Autodesk Inventor part; units mm, degrees
(part 2 of 2)
sketch "Sketch17" plane through (0, 22.225, 0) normal (0, 1, 0) x (1, 0, 0)
  line L0 (-762.5068, 1886.6652) -> (209.7128, 1886.6652) construction
  line L1 (209.7128, 1886.6652) -> (209.7128, -25.5438) construction
  line L2 (209.7128, -25.5438) -> (-762.5068, -25.5438) construction
  line L3 (-762.5068, -25.5438) -> (-762.5068, 1886.6652) construction
  line L4 (-762.5068, 1886.6652) -> (209.7128, 1886.6652) construction
  line L5 (209.7128, 1886.6652) -> (209.7128, -25.5438) construction
  line L6 (209.7128, -25.5438) -> (-762.5068, -25.5438) construction
  line L7 (-762.5068, -25.5438) -> (-762.5068, 1886.6652) construction
  point P0 (0, 0)
  point P1 (0, 0)
  point P2 (0, 0)
  constraints: 4 other
decal "Decal2"
sketch "Sketch18" plane through (0, 22.225, 0) normal (0, 1, 0) x (1, 0, 0)
  line L0 (-762.5068, 1886.6652) -> (209.7128, 1886.6652) construction
  line L1 (209.7128, 1886.6652) -> (209.7128, -25.5438) construction
  line L2 (209.7128, -25.5438) -> (-762.5068, -25.5438) construction
  line L3 (-762.5068, -25.5438) -> (-762.5068, 1886.6652) construction
  line L4 (-762.5068, 1886.6652) -> (209.7128, 1886.6652) construction
  line L5 (209.7128, 1886.6652) -> (209.7128, -25.5438) construction
  line L6 (209.7128, -25.5438) -> (-762.5068, -25.5438) construction
  line L7 (-762.5068, -25.5438) -> (-762.5068, 1886.6652) construction
  point P0 (0, 0)
  point P1 (0, 0)
  point P2 (0, 0)
  constraints: 4 other
decal "Decal3"
decal "Decal4"
decal "Decal5"
decal "Decal6"
decal "Decal7"
decal "Decal8"
decal "Decal9"
body "Solid1"
